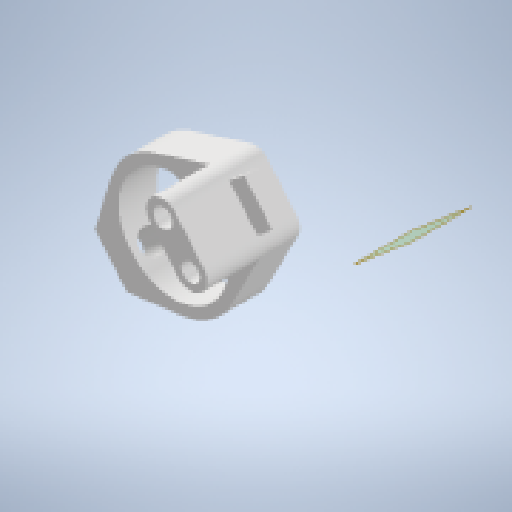
# Autodesk Inventor part: marker_cerret
Saved by Autodesk Inventor 2024 (Build 280153000, 153)
## iProperties
Created: 2026-02-15
Part Number: marker_cerret
Material: Generic
Document SubType Name: Modeling
Designer: SEMEN
Density: 1 g/cm^3
Appearance: Default
Author: SEMEN
Autodesk Inventor part; units mm, degrees
ref_plane "YZ Plane" through (0, 0, 0) normal (1, 0, 0) x (0, 1, 0)
ref_plane "XZ Plane" through (0, 0, 0) normal (0, 1, 0) x (-1, 0, 0)
ref_plane "XY Plane" through (0, 0, 0) normal (0, 0, 1) x (1, 0, 0)
sketch "Sketch1" plane through (0, 0, 0) normal (0, 0, 1) x (1, 0, 0)
  circle A0 centre (83.2518, -42.1897) radius 1.5 projected
  circle A1 centre (88.3962, -48.3162) radius 1.5 projected
  circle A2 centre (75.2518, -54.1305) radius 10 projected
  arc A3 (71.6612, -42.6802) -> (85.9084, -59.6473) centre (75.2518, -54.1305) ccw
  arc A4 (85.5492, -40.2605) -> (82.3541, -39.3271) centre (83.2518, -42.1897) ccw
  arc A5 (91.0604, -49.6954) -> (90.6937, -46.387) centre (88.3962, -48.3162) ccw
  line L0 (71.6612, -42.6802) -> (82.3541, -39.3271)
  line L1 (91.0604, -49.6954) -> (85.9084, -59.6473)
  line L2 (85.5492, -40.2605) -> (90.6937, -46.387)
  circle A6 centre (83.2518, -42.1897) radius 1.75
  circle A7 centre (88.3962, -48.3162) radius 1.7
  line L3 (88.1215, -43.3238) -> (66.062, -61.8472) construction
  line L4 (82.9099, -47.6999) -> (85.0453, -56.1521)
  line L5 (82.9099, -47.6999) -> (74.9544, -44.1349)
  circle A8 centre (75.2518, -54.1305) radius 9 construction
  line L6 (60.8256, -60.2763) -> (66.7035, -67.2763)
  line L7 (60.8256, -60.2763) -> (63.7758, -50.6232)
  line L8 (66.7035, -67.2763) -> (76.7214, -66.0401)
  point P0 (0, 0)
  dimension "d0" = 24
  dimension "d1" = 6
  dimension "d2" = 6
  dimension "d3" = 3.5
  dimension "d4" = 3.4
  dimension "d5" = 18
  dimension "d8" = 15
  dimension "d9" = 7
  constraints: 18 end point, 12 point on circle, 9 tangent, 6 centre point, 6 coincident, 1 midpoint, 1 parallel, 1 perpendicular, 1 point on line, 1 symmetric about line, 1 other
  measures "d0" diameter of A3
  measures "d1" diameter of A4
  measures "d2" diameter of A5
  measures "d3" diameter of A6
  measures "d4" diameter of A7
  measures "d5" diameter of A8
  measures "d8" distance from line of L6 A2.centre
  measures "d9" vertical distance of L6.end L6.start
extrude "Extrusion1" add sketch "Sketch1" along normal blind 9 contours A2 L4 | L5 A2 | L0 A4 L2 A5 L1 A3 | A3 L8 L6 L7
sketch "Sketch2" plane through (66.7035, -67.2763, 0) normal (-0.7658175, -0.643058, 0) x (0, 0, 1)
  line L0 (9, 9.1406) -> (9, 0) projected
  line L1 (9, 4.5703) -> (0, 4.5703) construction
  line L2 (0, 9.1406) -> (0, 0) projected
  line L3 (0, 9.1406) -> (9, 9.1406) projected
  line L4 (4.5, 9.1406) -> (4.5, 0) construction
  line L5 (0, 0) -> (9, 0) projected
  point P0 (0, 94.4156)
  point P1 (4.5, 4.5703)
  constraints: 5 midpoint, 4 end point
hole "Hole1" at (63.7645, -63.7763, 4.5) direction (0.7658175, 0.643058, 0) diameter 4.6 depth 8
ref_plane "Work Plane1" through (122.4886, -30.1352, -3.9205) normal (0.643058, -0.7658175, 0) x (0, 0, 1)
sketch "Sketch3" plane through (122.4886, -30.1352, -3.9205) normal (0.643058, -0.7658175, 0) x (0, 0, 1)
  line L0 (3.9205, 34.8) -> (12.9205, 34.8) projected
  line L1 (8.4716, 29.3) -> (8.4716, 32.8) projected
  line L2 (8.4716, 32.8) -> (8.4716, 33.3)
  line L3 (3.9205, 34.8) -> (12.9205, 34.8) projected
  line L4 (8.4716, 34.8) -> (9.4716, 33.05)
  line L5 (9.4716, 33.05) -> (8.4716, 31.3)
  line L6 (8.4716, 31.3) -> (12.9205, 31.3)
  line L7 (12.9205, 31.3) -> (12.9205, 34.8)
  line L8 (8.4716, 33.05) -> (10.4716, 33.05) construction
  point P0 (3.9205, 74.4253)
  dimension "d17" = 0.5
  dimension "d18" = 1
  constraints: 12 end point, 2 horizontal, 2 midpoint, 2 point on line, 1 perpendicular, 1 vertical, 2 other
  measures "d17" distance of L1.end L2.end
  measures "d18" distance from line of L2 L4.end
extrude "Extrusion2" add sketch "Sketch3" against normal blind 16
sketch "Sketch4" plane through (122.4886, -30.1352, -3.9205) normal (0.643058, -0.7658175, 0) x (0.7658175, 0.643058, 0)
  line L0 (-34.8, 12.9205) -> (-34.8, 8.4716) projected
  line L1 (-34.8, 8.4716) -> (-33.05, 9.4716) projected
  line L2 (-33.05, 9.4716) -> (-31.3, 8.4716) projected
  line L3 (-31.3, 8.4716) -> (-31.3, 12.9205) projected
  line L4 (-31.3, 12.9205) -> (-34.8, 12.9205) projected
  point P0 (-74.4253, 3.9205)
extrude "Extrusion3" cut sketch "Sketch4" against normal blind 8
sketch "Sketch5" plane through (0, 0, 9) normal (0, 0, 1) x (1, 0, 0)
  circle A0 centre (83.2518, -42.1897) radius 1.75 projected
  circle A1 centre (83.2518, -42.1897) radius 1.75 projected
  circle A2 centre (88.3962, -48.3162) radius 1.7 projected
  circle A3 centre (88.3962, -48.3162) radius 1.7 projected
  circle A4 centre (88.3962, -48.3162) radius 3
  circle A5 centre (83.2518, -42.1897) radius 3
  line L0 (85.5492, -40.2605) -> (90.6937, -46.387)
  line L1 (80.9543, -44.1188) -> (86.0988, -50.2454)
  point P0 (0, 0)
  dimension "d23" = 6
  dimension "d24" = 6
  constraints: 4 end point, 4 point on circle, 4 tangent, 2 centre point, 2 coincident
  measures "d23" diameter of A5
  measures "d24" diameter of A4
extrude "Extrusion4" add sketch "Sketch5" along normal blind 10
body "Solid1"
